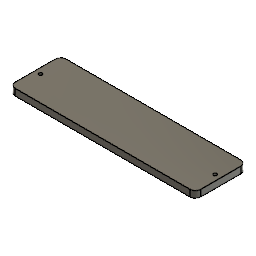
Specimen_Rack_v0 (Autodesk Fusion 360 design; units mm, degrees)
Autodesk Fusion 360 part; units mm, degrees
note: some values were not read from the file. Chosen so that the rebuilt part matches the saved one: which face or edge a step refers to; that a step has no effect; which pieces of a blend or face edit are solid.
sketch "Sketch1" plane through (0, 0, 0) normal (0, 1, 0) x (1, 0, 0) in component "Top_Layer"
  line L0 (0, 0) -> (250, 0)
  line L1 (250, 0) -> (250, 78)
  line L2 (250, 78) -> (0, 78)
  line L3 (0, 78) -> (0, 0)
  line L4 (0, 39) -> (250, 39) construction
  line L5 (0, 78) -> (0, 75) construction
  line L6 (0, 0) -> (0, 3) construction
  line L7 (0, 3) -> (250, 3) construction
  line L8 (0, 75) -> (250, 75) construction
  line L9 (250, 75) -> (247, 75) construction
  line L10 (247, 75) -> (247, 3) construction
  line L11 (0, 3) -> (3, 3) construction
  line L12 (3, 3) -> (3, 75) construction
  circle A0 centre (5.4622, 38.5669) radius 2.5
  circle A1 centre (244.5, 39) radius 2.5
  line L13 (242, 39) -> (237, 39) construction
  line L14 (7.9244, 39) -> (12.9244, 39) construction
  circle A2 centre (211.5, 39) radius 25.5
  circle A3 centre (38.4244, 39) radius 25.5
  line L15 (63.9244, 39) -> (73.9244, 39) construction
  line L16 (186, 39) -> (176, 39) construction
  circle A4 centre (89.4244, 39) radius 15.5
  circle A5 centre (160.5, 39) radius 15.5
  line L17 (104.9244, 39) -> (145, 39) construction
  circle A6 centre (124.9622, 39) radius 15.5
  dimension "d1" = 250
  dimension "d2" = 78
  dimension "d3" = 3
  dimension "d4" = 3
  dimension "d5" = 3
  dimension "d6" = 3
  dimension "d7" = 5
  dimension "d8" = 5
  dimension "d9" = 5
  dimension "d10" = 5
  dimension "d11" = 51
  dimension "d12" = 51
  dimension "d13" = 10
  dimension "d14" = 10
  dimension "d15" = 31
  dimension "d16" = 31
  dimension "d17" = 31
  constraint horizontal L0
  constraint vertical L1
  constraint horizontal L2
  constraint vertical L3
  constraint coincident L0.start L3.end
  constraint midpoint L3 L4.start
  constraint midpoint L1 L4.end
  constraint perpendicular L2 L5
  constraint perpendicular L0 L6
  constraint coincident L1 L7.end
  constraint perpendicular L1 L7
  constraint coincident L1 L8.end
  constraint perpendicular L1 L8
  constraint perpendicular L1 L9
  constraint coincident L7 L10.end
  constraint perpendicular L7 L10
  constraint perpendicular L6 L11
  constraint perpendicular L7 L12
  constraint coincident A1 L13.start
  constraint coincident L4 L13.start
  constraint coincident L4 L13.end
  constraint coincident A0 L14.start
  constraint coincident L4 L14.start
  constraint perpendicular L3 L14
  constraint coincident L13.end A2
  constraint coincident L14.end A3
  constraint coincident A3 L15.start
  constraint coincident L4 L15.start
  constraint parallel L4 L15
  constraint coincident A2 L16.start
  constraint coincident L4 L16.start
  constraint parallel L4 L16
  constraint coincident L15.end A4
  constraint coincident L16.end A5
  constraint coincident A4 L17.start
  constraint coincident L4 L17.start
  constraint coincident A5 L17.end
  constraint coincident L4 L17.end
  constraint midpoint L17 A6.centre
  measures "d1" distance of L0.start L0.end
  measures "d2" distance of L0.start L2.end
  measures "d3" distance of L2.end L5.end
  measures "d4" distance of L0.start L6.end
  measures "d5" distance of L8.end L9.end
  measures "d6" distance of L6.end L11.end
  measures "d7" diameter of A0
  measures "d8" diameter of A1
  measures "d9" distance of L13.start L13.end
  measures "d10" distance of L14.start L14.end
  measures "d11" diameter of A2
  measures "d12" diameter of A3
  measures "d13" distance of L15.start L15.end
  measures "d14" distance of L16.start L16.end
  measures "d15" diameter of A4
  measures "d16" diameter of A5
  measures "d17" diameter of A6
extrude "Extrude1" add sketch "Sketch1" along normal blind 5 contours A0 | A1 makes body 1 at (7.9591, 3.3333, -38.4423) makes body 2 at (245.1771, 3.3333, -41.4066) in component "Top_Layer"
extrude "Extrude2" add sketch "Sketch1" along normal blind 10 bodies 1 2 in component "Top_Layer"
move_face "MoveFace1" to x (1, 0, 0) y (0, 1, 0) z (0, 0, 1) at (50, 0, 0) 2 faces at (250, 3.3333, -26) (245.2962, 6.6667, -41.3698) on bodies 1 in component "Top_Layer"
move_face "MoveFace2" to x (1, 0, 0) y (0, 1, 0) z (0, 0, 1) at (5.462, 0, 0) 2 faces at (175.923, 3.3333, -37.4567) (236.8733, 3.3333, -36.461) on bodies 1 in component "Top_Layer"
move_face "MoveFace3" to x (1, 0, 0) y (0, 1, 0) z (0, 0, 1) at (5.462, 0, 0) 3 faces at (140.4429, 6.6667, -38.2274) (181.385, 3.3333, -37.4567) (242.3353, 3.3333, -36.461) on bodies 1 in component "Top_Layer"
fillet "Fillet1" radius 8 4 edges at (0, 5, -78) (0, 5, 0) (300, 5, 0) (300, 5, -78) on bodies 1 in component "Top_Layer"
sketch "Sketch2" plane through (0, 10, 0) normal (0, 1, 0) x (-1, 0, 0) in component "Top_Layer"
  circle A0 centre (-5.4622, -38.5669) radius 2.5
  circle A1 centre (-38.4244, -39) radius 25.5
  circle A2 centre (-171.424, -39) radius 15.5
  circle A3 centre (-130.4242, -39) radius 15.5
  circle A4 centre (-89.4244, -39) radius 15.5
  circle A5 centre (-294.5, -39) radius 2.5
  circle A6 centre (-222.424, -39) radius 25.5
  arc A7 (-300, -70) -> (-292, -78) centre (-292, -70) ccw
  line L0 (-292, -78) -> (-8, -78)
  arc A8 (-8, -78) -> (0, -70) centre (-8, -70) ccw
  line L1 (0, -70) -> (0, -8)
  arc A9 (0, -8) -> (-8, 0) centre (-8, -8) ccw
  arc A10 (-292, 0) -> (-300, -8) centre (-292, -8) ccw
  line L2 (-300, -8) -> (-300, -70)
  line L3 (-247.9239, -38.9231) -> (-292.0012, -38.9231) construction
  line L4 (-222.424, -39) -> (-171.424, -39) construction
  line L5 (-171.424, -39) -> (-130.4242, -39) construction
  line L6 (-130.4242, -39) -> (-89.4244, -39) construction
  line L7 (-89.4244, -39) -> (-38.4244, -39) construction
  line L8 (-73.9244, -39) -> (-63.9244, -39) construction
  line L9 (-104.9244, -39) -> (-114.9242, -39) construction
  line L10 (-145.9242, -39) -> (-155.924, -39) construction
  line L11 (-186.924, -39) -> (-196.924, -39) construction
  line L12 (-191.924, -39) -> (-191.924, 0) construction
  line L13 (-191.924, 0) -> (-191.924, -6) construction
  line L14 (-68.9244, -39) -> (-68.9244, -78) construction
  line L15 (-68.9244, -78) -> (-68.9244, -72) construction
  line L16 (-191.924, -6) -> (-68.9244, -6) construction
  line L17 (-68.9244, -6) -> (-68.9244, -72) construction
  line L18 (-68.9244, -72) -> (-191.924, -72) construction
  line L19 (-191.924, -72) -> (-191.924, -6) construction
  line L20 (-150.9241, -39) -> (-150.9241, -72) construction
  line L21 (-150.9241, -39) -> (-150.9241, -6) construction
  line L22 (-109.9243, -39) -> (-109.9243, -72) construction
  line L23 (-109.9243, -39) -> (-109.9243, -6) construction
  line L24 (-171.424, -39) -> (-171.424, -23.5) construction
  line L25 (-171.424, -23.5) -> (-171.424, -17.5) construction
  line L26 (-171.424, -17.5) -> (-68.9244, -17.5) construction
  line L27 (-171.424, -39) -> (-171.424, -54.5) construction
  line L28 (-171.424, -54.5) -> (-171.424, -60.5) construction
  line L29 (-171.424, -60.5) -> (-68.9244, -60.4734) construction
  circle A11 centre (-150.9241, -65.5) radius 6.5
  circle A12 centre (-150.9241, -12.5) radius 6.5
  circle A13 centre (-109.9243, -12.5) radius 6.5
  circle A14 centre (-68.9244, -12.5) radius 6.5
  circle A15 centre (-68.9244, -65.5) radius 6.5
  circle A16 centre (-109.926, -65.5) radius 6.5
  circle A17 centre (-191.924, -65.5) radius 6.5
  circle A18 centre (-191.924, -12.5) radius 6.5
  dimension "d32" = 6
  dimension "d33" = 6
  dimension "d34" = 6
  dimension "d35" = 6
  dimension "d36" = 13
  dimension "d37" = 13
  dimension "d38" = 13
  dimension "d39" = 13
  dimension "d40" = 13
  dimension "d41" = 13
  dimension "d42" = 13
  dimension "d43" = 13
  constraint coincident A6 L3.start
  constraint coincident A5 L3.end
  constraint horizontal L3
  constraint coincident A6.centre L4.start
  constraint coincident A2.centre L4.end
  constraint coincident A3.centre L5.end
  constraint coincident A4.centre L6.end
  constraint coincident A1.centre L7.end
  constraint coincident A4 L8.start
  constraint coincident L7 L8.start
  constraint midpoint L7 L8.end
  constraint coincident A4 L9.start
  constraint coincident L6 L9.start
  constraint coincident L6 L9.end
  constraint coincident A3 L9.end
  constraint coincident A3 L10.start
  constraint coincident L5 L10.start
  constraint coincident A2 L10.end
  constraint coincident L5 L10.end
  constraint coincident A2 L11.start
  constraint coincident L4 L11.start
  constraint midpoint L4 L11.end
  constraint midpoint L11 L12.start
  constraint midpoint L8 L14.start
  constraint coincident L0 L14.end
  constraint perpendicular L0 L14
  constraint perpendicular L0 L15
  constraint horizontal L16
  constraint vertical L17
  constraint horizontal L18
  constraint vertical L19
  constraint midpoint L5 L20.start
  constraint coincident L18 L20.end
  constraint perpendicular L18 L20
  constraint coincident L16 L21.end
  constraint perpendicular L16 L21
  constraint midpoint L6 L22.start
  constraint coincident L18 L22.end
  constraint perpendicular L18 L22
  constraint coincident L16 L23.end
  constraint perpendicular L16 L23
  constraint coincident A2 L24.end
  constraint perpendicular L4 L24
  constraint parallel L24 L25
  constraint coincident L17 L26.end
  constraint perpendicular L17 L26
  constraint coincident A2 L27.end
  constraint perpendicular L4 L27
  constraint parallel L27 L28
  constraint coincident L17 L29.end
  constraint coincident L20.end A11
  constraint coincident L21.end A12
  constraint coincident L23.end A13
  constraint coincident L16.end A14
  constraint coincident L15.end A15
  constraint coincident L22.end A16
  constraint coincident L18.end A17
  constraint coincident L13.end A18
  measures "d32" distance of L12.end L13.end
  measures "d33" distance of L14.end L15.end
  measures "d34" distance of L24.end L25.end
  measures "d35" distance of L27.end L28.end
  measures "d36" diameter of A11
  measures "d37" diameter of A12
  measures "d38" diameter of A13
  measures "d39" diameter of A14
  measures "d40" diameter of A15
  measures "d41" diameter of A16
  measures "d42" diameter of A17
  measures "d43" diameter of A18
extrude "Extrude3" cut sketch "Sketch2" against normal blind 10 contours A11 | A12 | A13 | A14 | A15 | A16 | A17 | A18 bodies 1 in component "Top_Layer"
sketch "Sketch3" plane through (0, 10, 0) normal (0, 1, 0) x (-1, 0, 0) in component "Top_Layer"
move_face "MoveFace4" to x (1, 0, 0) y (0, 1, 0) z (0, 0, 1) at (-34.07, 0, 0) 7 faces at (282.6413, 0, -39) (297.7899, 6.6667, -75.5206) (276.6758, 10, -56.2406) (300, 3.3333, -28.6667) (297.7899, 3.3333, -2.4794) (294.9341, 6.6667, -41.462) (295.1109, 5, -38.1848) on bodies 1 in component "Top_Layer"
move_face "MoveFace5" to x (1, 0, 0) y (0, 1, 0) z (0, 0, 1) at (-0.006, 0, 0) 2 faces at (265.93, 3.3333, -28.6667) (260.7409, 8.3333, -41.4806) on bodies 1 in component "Top_Layer"
move_face "MoveFace6" by (3, 0, 0) 1 faces at (265.93, 3.3333, -28.6667) on bodies 1 in component "Top_Layer"
move_face "MoveFace7" to x (1, 0, 0) y (0, 1, 0) z (0, 0, 1) at (-5.025, 0, 0) 5 faces at (0.0091, 3.3333, -70.3807) (7.6193, 3.3333, -0.0091) (0, 3.3333, -49.3333) (7.9591, 6.6667, -38.6915) (4.6036, 5, -39.1523) on bodies 1 in component "Top_Layer"
move_face "MoveFace8" to x (1, 0, 0) y (0, 1, 0) z (0, 0, 1) at (-0.005, 0, 0) 2 faces at (2.9341, 6.6667, -38.6915) (-5.025, 5, -64.039) on bodies 1 in component "Top_Layer"
move_face "MoveFace9" by (-3.038, 0, 0) 1 faces at (-5.025, 5, -64.039) on bodies 1 in component "Top_Layer"
sketch "Sketch4" plane through (0, 10, 0) normal (0, 1, 0) x (-1, 0, 0) in component "Top_Layer"
  arc A0 (8.068, -8) -> (0.068, 0) centre (0.068, -8) ccw
  line L0 (0.068, 0) -> (-260.924, 0)
  arc A1 (-260.924, 0) -> (-268.924, -8) centre (-260.924, -8) ccw
  line L1 (-268.924, -8) -> (-268.924, -70)
  arc A2 (-268.924, -70) -> (-260.924, -78) centre (-260.924, -70) ccw
  line L2 (-260.924, -78) -> (0.068, -78)
  arc A3 (0.068, -78) -> (8.068, -70) centre (0.068, -70) ccw
  line L3 (8.068, -70) -> (8.068, -8)
  circle A4 centre (-109.9243, -12.5) radius 6.5
  circle A5 centre (-191.924, -12.5) radius 6.5
  circle A6 centre (-150.9241, -12.5) radius 6.5
  circle A7 centre (-68.9244, -12.5) radius 6.5
  circle A8 centre (-150.9241, -65.5) radius 6.5
  circle A9 centre (-191.924, -65.5) radius 6.5
  circle A10 centre (-109.926, -65.5) radius 6.5
  circle A11 centre (-68.9244, -65.5) radius 6.5
  circle A12 centre (-0.4322, -38.5669) radius 2.5
  circle A13 centre (-38.4244, -39) radius 25.5
  circle A14 centre (-171.424, -39) radius 15.5
  circle A15 centre (-130.4242, -39) radius 15.5
  circle A16 centre (-89.4244, -39) radius 15.5
  circle A17 centre (-260.424, -39) radius 2.5
  circle A18 centre (-222.424, -39) radius 25.5
  line L4 (-260.424, -39) -> (-247.924, -39) construction
  line L5 (-191.924, -65.5) -> (-191.924, -72) construction
  line L6 (-191.924, -72) -> (-268.67, -72) construction
  line L7 (-254.174, -39) -> (-254.174, -72) construction
  line L8 (-254.174, -39) -> (-191.9575, -39) construction
  line L9 (-191.9575, -39) -> (-191.9575, -6.0001) construction
  line L10 (-191.9575, -6.0001) -> (-254.174, -6.0001) construction
  line L11 (-254.174, -6.0001) -> (-254.174, -39) construction
  circle A19 centre (-254.174, -12.5001) radius 6.5
  circle A20 centre (-254.174, -65.5) radius 6.5
  dimension "d64" = 13
  dimension "d65" = 13
  constraint coincident A17.centre L4.start
  constraint coincident A18 L4.end
  constraint perpendicular L1 L4
  constraint coincident A9.centre L5.start
  constraint coincident A9 L5.end
  constraint vertical L5
  constraint coincident A2 L6.end
  constraint tangent A9 L6
  constraint midpoint L4 L7.start
  constraint coincident L6 L7.end
  constraint perpendicular L6 L7
  constraint horizontal L8
  constraint vertical L9
  constraint horizontal L10
  constraint vertical L11
  constraint coincident A5 L9.end
  constraint coincident L10.end A19
  constraint coincident L7.end A20
  measures "d64" diameter of A19
  measures "d65" diameter of A20
extrude "Extrude4" cut sketch "Sketch4" against normal blind 13 contours A19 | A20 bodies 1 in component "Top_Layer"
sketch "Sketch5" plane through (0, 10, 0) normal (0, 1, 0) x (-1, 0, 0) in component "Top_Layer"
  circle A0 centre (-254.174, -65.5) radius 6.5
  circle A1 centre (-254.174, -12.5001) radius 6.5
  arc A2 (8.068, -8) -> (0.068, 0) centre (0.068, -8) ccw
  line L0 (0.068, 0) -> (-260.924, 0)
  arc A3 (-260.924, 0) -> (-268.924, -8) centre (-260.924, -8) ccw
  line L1 (-268.924, -8) -> (-268.924, -70)
  arc A4 (-268.924, -70) -> (-260.924, -78) centre (-260.924, -70) ccw
  line L2 (-260.924, -78) -> (0.068, -78)
  arc A5 (0.068, -78) -> (8.068, -70) centre (0.068, -70) ccw
  line L3 (8.068, -70) -> (8.068, -8)
  circle A6 centre (-109.9243, -12.5) radius 6.5
  circle A7 centre (-191.924, -12.5) radius 6.5
  circle A8 centre (-150.9241, -12.5) radius 6.5
  circle A9 centre (-68.9244, -12.5) radius 6.5
  circle A10 centre (-150.9241, -65.5) radius 6.5
  circle A11 centre (-191.924, -65.5) radius 6.5
  circle A12 centre (-109.926, -65.5) radius 6.5
  circle A13 centre (-68.9244, -65.5) radius 6.5
  circle A14 centre (-0.4322, -38.5669) radius 2.5
  circle A15 centre (-38.4244, -39) radius 25.5
  circle A16 centre (-171.424, -39) radius 15.5
  circle A17 centre (-130.4242, -39) radius 15.5
  circle A18 centre (-89.4244, -39) radius 15.5
  circle A19 centre (-260.424, -39) radius 2.5
  circle A20 centre (-222.424, -39) radius 25.5
  line L4 (-0.4322, -38.5669) -> (-2.9322, -38.5669) construction
  line L5 (-2.9322, -38.5669) -> (-12.9281, -38.5669) construction
  line L6 (-69.0119, -6.0006) -> (-66.2573, -5.9635) construction
  line L7 (-66.2573, -5.9635) -> (7.8045, -5.9635) construction
  line L8 (-7.9301, -38.5669) -> (-7.9301, -5.9635) construction
  line L9 (-7.9301, -5.9635) -> (-68.6986, -5.9635) construction
  line L10 (-68.6986, -5.9635) -> (-68.6986, -71.9961) construction
  line L11 (-68.6986, -71.9961) -> (-7.9301, -71.9961) construction
  line L12 (-7.9301, -71.9961) -> (-7.9301, -5.9635) construction
  circle A21 centre (-7.9301, -12.4635) radius 6.5
  circle A22 centre (-7.9301, -65.4961) radius 6.5
  dimension "d68" = 13
  dimension "d69" = 13
  constraint coincident A14.centre L4.start
  constraint coincident A14 L4.end
  constraint horizontal L4
  constraint coincident A15 L5.end
  constraint parallel L4 L5
  constraint coincident A9 L6.start
  constraint tangent A9 L6
  constraint coincident A2 L7.end
  constraint parallel L0 L7
  constraint midpoint L5 L8.start
  constraint coincident L7 L8.end
  constraint perpendicular L7 L8
  constraint horizontal L9
  constraint vertical L10
  constraint horizontal L11
  constraint vertical L12
  constraint coincident A13 L10.end
  constraint coincident L8.end A21
  constraint coincident L11.end A22
  measures "d68" diameter of A21
  measures "d69" diameter of A22
extrude "Extrude5" cut sketch "Sketch5" against normal blind 10 contours A21 | A22 bodies 1 in component "Top_Layer"
move_face "MoveFace10" to x (1, 0, 0) y (0, 1, 0) z (0, 0, 1) at (0, 0, 2) 6 faces at (1.4382, 3.3333, -65.8201) (62.4325, 3.3333, -65.824) (103.4341, 3.3333, -65.824) (144.4322, 3.3333, -65.824) (185.4563, 6.6667, -66.1472) (258.475, 6.6667, -60.6264) on bodies 1 in component "Top_Layer"
move_face "MoveFace11" to x (1, 0, 0) y (0, 1, 0) z (0, 0, 1) at (0, 0, -2) 6 faces at (1.4382, 3.3333, -12.7875) (62.4325, 3.3333, -12.824) (103.4324, 3.3333, -12.824) (144.4322, 3.3333, -12.824) (185.4563, 6.6667, -13.1472) (258.475, 6.6667, -7.6265) on bodies 1 in component "Top_Layer"
sketch "Sketch1 (2)" plane through (0, 0, 0) normal (0, 1, 0) x (1, 0, 0) in component "Bottom_Layer"
  line L0 (0, 0) -> (250, 0)
  line L1 (250, 0) -> (250, 78)
  line L2 (250, 78) -> (0, 78)
  line L3 (0, 78) -> (0, 0)
  line L4 (0, 39) -> (250, 39) construction
  line L5 (0, 78) -> (0, 75) construction
  line L6 (0, 0) -> (0, 3) construction
  line L7 (0, 3) -> (250, 3) construction
  line L8 (0, 75) -> (250, 75) construction
  line L9 (250, 75) -> (247, 75) construction
  line L10 (247, 75) -> (247, 3) construction
  line L11 (0, 3) -> (3, 3) construction
  line L12 (3, 3) -> (3, 75) construction
  circle A0 centre (5.4622, 38.5669) radius 2.5
  circle A1 centre (244.5, 39) radius 2.5
  line L13 (242, 39) -> (237, 39) construction
  line L14 (7.9244, 39) -> (12.9244, 39) construction
  circle A2 centre (211.5, 39) radius 25.5
  circle A3 centre (38.4244, 39) radius 25.5
  line L15 (63.9244, 39) -> (73.9244, 39) construction
  line L16 (186, 39) -> (176, 39) construction
  circle A4 centre (89.4244, 39) radius 15.5
  circle A5 centre (160.5, 39) radius 15.5
  line L17 (104.9244, 39) -> (145, 39) construction
  circle A6 centre (124.9622, 39) radius 15.5
  dimension "d1_1" = 250
  dimension "d2_1" = 78
  dimension "d3_1" = 3
  dimension "d4_1" = 3
  dimension "d5_1" = 3
  dimension "d6_1" = 3
  dimension "d7_1" = 5
  dimension "d8_1" = 5
  dimension "d9_1" = 5
  dimension "d10_1" = 5
  dimension "d11_1" = 51
  dimension "d12_1" = 51
  dimension "d13_1" = 10
  dimension "d14_1" = 10
  dimension "d15_1" = 31
  dimension "d16_1" = 31
  dimension "d17_1" = 31
  constraint horizontal L0
  constraint vertical L1
  constraint horizontal L2
  constraint vertical L3
  constraint coincident L0.start L3.end
  constraint midpoint L3 L4.start
  constraint midpoint L1 L4.end
  constraint perpendicular L2 L5
  constraint perpendicular L0 L6
  constraint coincident L1 L7.end
  constraint perpendicular L1 L7
  constraint coincident L1 L8.end
  constraint perpendicular L1 L8
  constraint perpendicular L1 L9
  constraint coincident L7 L10.end
  constraint perpendicular L7 L10
  constraint perpendicular L6 L11
  constraint perpendicular L7 L12
  constraint coincident A1 L13.start
  constraint coincident L4 L13.start
  constraint coincident L4 L13.end
  constraint coincident A0 L14.start
  constraint coincident L4 L14.start
  constraint perpendicular L3 L14
  constraint coincident L13.end A2
  constraint coincident L14.end A3
  constraint coincident A3 L15.start
  constraint coincident L4 L15.start
  constraint parallel L4 L15
  constraint coincident A2 L16.start
  constraint coincident L4 L16.start
  constraint parallel L4 L16
  constraint coincident L15.end A4
  constraint coincident L16.end A5
  constraint coincident A4 L17.start
  constraint coincident L4 L17.start
  constraint coincident A5 L17.end
  constraint coincident L4 L17.end
  constraint midpoint L17 A6.centre
  measures "d1_1" distance of L0.start L0.end
  measures "d2_1" distance of L0.start L2.end
  measures "d3_1" distance of L2.end L5.end
  measures "d4_1" distance of L0.start L6.end
  measures "d5_1" distance of L8.end L9.end
  measures "d6_1" distance of L6.end L11.end
  measures "d7_1" diameter of A0
  measures "d8_1" diameter of A1
  measures "d9_1" distance of L13.start L13.end
  measures "d10_1" distance of L14.start L14.end
  measures "d11_1" diameter of A2
  measures "d12_1" diameter of A3
  measures "d13_1" distance of L15.start L15.end
  measures "d14_1" distance of L16.start L16.end
  measures "d15_1" diameter of A4
  measures "d16_1" diameter of A5
  measures "d17_1" diameter of A6
extrude "Extrude1'" add sketch "Sketch1 (2)" along normal blind 5 separate body contours A0 | A1 makes body 3 at (7.9591, 3.3333, -38.4423) makes body 4 at (245.1771, 3.3333, -41.4066) in component "Bottom_Layer"
extrude "Extrude2'" add sketch "Sketch1 (2)" along normal blind 10 bodies 3 4 in component "Bottom_Layer"
move_face "MoveFace1'" to x (1, 0, 0) y (0, 1, 0) z (0, 0, 1) at (50, 0, 0) 2 faces at (250, 3.3333, -26) (245.2962, 6.6667, -41.3698) on bodies 3 in component "Bottom_Layer"
move_face "MoveFace2'" to x (1, 0, 0) y (0, 1, 0) z (0, 0, 1) at (5.462, 0, 0) 2 faces at (175.923, 3.3333, -37.4567) (236.8733, 3.3333, -36.461) on bodies 3 in component "Bottom_Layer"
move_face "MoveFace3'" to x (1, 0, 0) y (0, 1, 0) z (0, 0, 1) at (5.462, 0, 0) 3 faces at (140.4429, 6.6667, -38.2274) (181.385, 3.3333, -37.4567) (242.3353, 3.3333, -36.461) on bodies 3 in component "Bottom_Layer"
fillet "Fillet1'" radius 8 4 edges at (0, 5, -78) (0, 5, 0) (300, 5, 0) (300, 5, -78) on bodies 3 in component "Bottom_Layer"
sketch "Sketch2 (2)" plane through (0, 10, 0) normal (0, 1, 0) x (-1, 0, 0) in component "Bottom_Layer"
  circle A0 centre (-5.4622, -38.5669) radius 2.5
  circle A1 centre (-38.4244, -39) radius 25.5
  circle A2 centre (-171.424, -39) radius 15.5
  circle A3 centre (-130.4242, -39) radius 15.5
  circle A4 centre (-89.4244, -39) radius 15.5
  circle A5 centre (-294.5, -39) radius 2.5
  circle A6 centre (-222.424, -39) radius 25.5
  arc A7 (-300, -70) -> (-292, -78) centre (-292, -70) ccw
  line L0 (-292, -78) -> (-8, -78)
  arc A8 (-8, -78) -> (0, -70) centre (-8, -70) ccw
  line L1 (0, -70) -> (0, -8)
  arc A9 (0, -8) -> (-8, 0) centre (-8, -8) ccw
  arc A10 (-292, 0) -> (-300, -8) centre (-292, -8) ccw
  line L2 (-300, -8) -> (-300, -70)
  line L3 (-247.9239, -38.9231) -> (-292.0012, -38.9231) construction
  line L4 (-222.424, -39) -> (-171.424, -39) construction
  line L5 (-171.424, -39) -> (-130.4242, -39) construction
  line L6 (-130.4242, -39) -> (-89.4244, -39) construction
  line L7 (-89.4244, -39) -> (-38.4244, -39) construction
  line L8 (-73.9244, -39) -> (-63.9244, -39) construction
  line L9 (-104.9244, -39) -> (-114.9242, -39) construction
  line L10 (-145.9242, -39) -> (-155.924, -39) construction
  line L11 (-186.924, -39) -> (-196.924, -39) construction
  line L12 (-191.924, -39) -> (-191.924, 0) construction
  line L13 (-191.924, 0) -> (-191.924, -6) construction
  line L14 (-68.9244, -39) -> (-68.9244, -78) construction
  line L15 (-68.9244, -78) -> (-68.9244, -72) construction
  line L16 (-191.924, -6) -> (-68.9244, -6) construction
  line L17 (-68.9244, -6) -> (-68.9244, -72) construction
  line L18 (-68.9244, -72) -> (-191.924, -72) construction
  line L19 (-191.924, -72) -> (-191.924, -6) construction
  line L20 (-150.9241, -39) -> (-150.9241, -72) construction
  line L21 (-150.9241, -39) -> (-150.9241, -6) construction
  line L22 (-109.9243, -39) -> (-109.9243, -72) construction
  line L23 (-109.9243, -39) -> (-109.9243, -6) construction
  line L24 (-171.424, -39) -> (-171.424, -23.5) construction
  line L25 (-171.424, -23.5) -> (-171.424, -17.5) construction
  line L26 (-171.424, -17.5) -> (-68.9244, -17.5) construction
  line L27 (-171.424, -39) -> (-171.424, -54.5) construction
  line L28 (-171.424, -54.5) -> (-171.424, -60.5) construction
  line L29 (-171.424, -60.5) -> (-68.9244, -60.4734) construction
  circle A11 centre (-150.9241, -65.5) radius 6.5
  circle A12 centre (-150.9241, -12.5) radius 6.5
  circle A13 centre (-109.9243, -12.5) radius 6.5
  circle A14 centre (-68.9244, -12.5) radius 6.5
  circle A15 centre (-68.9244, -65.5) radius 6.5
  circle A16 centre (-109.926, -65.5) radius 6.5
  circle A17 centre (-191.924, -65.5) radius 6.5
  circle A18 centre (-191.924, -12.5) radius 6.5
  dimension "d32_1" = 6
  dimension "d33_1" = 6
  dimension "d34_1" = 6
  dimension "d35_1" = 6
  dimension "d36_1" = 13
  dimension "d37_1" = 13
  dimension "d38_1" = 13
  dimension "d39_1" = 13
  dimension "d40_1" = 13
  dimension "d41_1" = 13
  dimension "d42_1" = 13
  dimension "d43_1" = 13
  constraint coincident A6 L3.start
  constraint coincident A5 L3.end
  constraint horizontal L3
  constraint coincident A6.centre L4.start
  constraint coincident A2.centre L4.end
  constraint coincident A3.centre L5.end
  constraint coincident A4.centre L6.end
  constraint coincident A1.centre L7.end
  constraint coincident A4 L8.start
  constraint coincident L7 L8.start
  constraint midpoint L7 L8.end
  constraint coincident A4 L9.start
  constraint coincident L6 L9.start
  constraint coincident L6 L9.end
  constraint coincident A3 L9.end
  constraint coincident A3 L10.start
  constraint coincident L5 L10.start
  constraint coincident A2 L10.end
  constraint coincident L5 L10.end
  constraint coincident A2 L11.start
  constraint coincident L4 L11.start
  constraint midpoint L4 L11.end
  constraint midpoint L11 L12.start
  constraint midpoint L8 L14.start
  constraint coincident L0 L14.end
  constraint perpendicular L0 L14
  constraint perpendicular L0 L15
  constraint horizontal L16
  constraint vertical L17
  constraint horizontal L18
  constraint vertical L19
  constraint midpoint L5 L20.start
  constraint coincident L18 L20.end
  constraint perpendicular L18 L20
  constraint coincident L16 L21.end
  constraint perpendicular L16 L21
  constraint midpoint L6 L22.start
  constraint coincident L18 L22.end
  constraint perpendicular L18 L22
  constraint coincident L16 L23.end
  constraint perpendicular L16 L23
  constraint coincident A2 L24.end
  constraint perpendicular L4 L24
  constraint parallel L24 L25
  constraint coincident L17 L26.end
  constraint perpendicular L17 L26
  constraint coincident A2 L27.end
  constraint perpendicular L4 L27
  constraint parallel L27 L28
  constraint coincident L17 L29.end
  constraint coincident L20.end A11
  constraint coincident L21.end A12
  constraint coincident L23.end A13
  constraint coincident L16.end A14
  constraint coincident L15.end A15
  constraint coincident L22.end A16
  constraint coincident L18.end A17
  constraint coincident L13.end A18
  measures "d32_1" distance of L12.end L13.end
  measures "d33_1" distance of L14.end L15.end
  measures "d34_1" distance of L24.end L25.end
  measures "d35_1" distance of L27.end L28.end
  measures "d36_1" diameter of A11
  measures "d37_1" diameter of A12
  measures "d38_1" diameter of A13
  measures "d39_1" diameter of A14
  measures "d40_1" diameter of A15
  measures "d41_1" diameter of A16
  measures "d42_1" diameter of A17
  measures "d43_1" diameter of A18
extrude "Extrude3'" cut sketch "Sketch2 (2)" against normal blind 10 contours A11 | A12 | A13 | A14 | A15 | A16 | A17 | A18 bodies 3 in component "Bottom_Layer"
sketch "Sketch3 (2)" plane through (0, 10, 0) normal (0, 1, 0) x (-1, 0, 0) in component "Bottom_Layer"
move_face "MoveFace4'" to x (1, 0, 0) y (0, 1, 0) z (0, 0, 1) at (-34.07, 0, 0) 7 faces at (282.6413, 0, -39) (297.7899, 6.6667, -75.5206) (276.6758, 10, -56.2406) (300, 3.3333, -28.6667) (297.7899, 3.3333, -2.4794) (294.9341, 6.6667, -41.462) (295.1109, 5, -38.1848) on bodies 3 in component "Bottom_Layer"
move_face "MoveFace5'" to x (1, 0, 0) y (0, 1, 0) z (0, 0, 1) at (-0.006, 0, 0) 2 faces at (265.93, 3.3333, -28.6667) (260.7409, 8.3333, -41.4806) on bodies 3 in component "Bottom_Layer"
move_face "MoveFace6'" by (3, 0, 0) 1 faces at (265.93, 3.3333, -28.6667) on bodies 3 in component "Bottom_Layer"
move_face "MoveFace7'" to x (1, 0, 0) y (0, 1, 0) z (0, 0, 1) at (-5.025, 0, 0) 5 faces at (0.0091, 3.3333, -70.3807) (7.6193, 3.3333, -0.0091) (0, 3.3333, -49.3333) (7.9591, 6.6667, -38.6915) (4.6036, 5, -39.1523) on bodies 3 in component "Bottom_Layer"
move_face "MoveFace8'" to x (1, 0, 0) y (0, 1, 0) z (0, 0, 1) at (-0.005, 0, 0) 2 faces at (2.9341, 6.6667, -38.6915) (-5.025, 5, -64.039) on bodies 3 in component "Bottom_Layer"
move_face "MoveFace9'" by (-3.038, 0, 0) 1 faces at (-5.025, 5, -64.039) on bodies 3 in component "Bottom_Layer"
sketch "Sketch4 (2)" plane through (0, 10, 0) normal (0, 1, 0) x (-1, 0, 0) in component "Bottom_Layer"
  arc A0 (8.068, -8) -> (0.068, 0) centre (0.068, -8) ccw
  line L0 (0.068, 0) -> (-260.924, 0)
  arc A1 (-260.924, 0) -> (-268.924, -8) centre (-260.924, -8) ccw
  line L1 (-268.924, -8) -> (-268.924, -70)
  arc A2 (-268.924, -70) -> (-260.924, -78) centre (-260.924, -70) ccw
  line L2 (-260.924, -78) -> (0.068, -78)
  arc A3 (0.068, -78) -> (8.068, -70) centre (0.068, -70) ccw
  line L3 (8.068, -70) -> (8.068, -8)
  circle A4 centre (-109.9243, -12.5) radius 6.5
  circle A5 centre (-191.924, -12.5) radius 6.5
  circle A6 centre (-150.9241, -12.5) radius 6.5
  circle A7 centre (-68.9244, -12.5) radius 6.5
  circle A8 centre (-150.9241, -65.5) radius 6.5
  circle A9 centre (-191.924, -65.5) radius 6.5
  circle A10 centre (-109.926, -65.5) radius 6.5
  circle A11 centre (-68.9244, -65.5) radius 6.5
  circle A12 centre (-0.4322, -38.5669) radius 2.5
  circle A13 centre (-38.4244, -39) radius 25.5
  circle A14 centre (-171.424, -39) radius 15.5
  circle A15 centre (-130.4242, -39) radius 15.5
  circle A16 centre (-89.4244, -39) radius 15.5
  circle A17 centre (-260.424, -39) radius 2.5
  circle A18 centre (-222.424, -39) radius 25.5
  line L4 (-260.424, -39) -> (-247.924, -39) construction
  line L5 (-191.924, -65.5) -> (-191.924, -72) construction
  line L6 (-191.924, -72) -> (-268.67, -72) construction
  line L7 (-254.174, -39) -> (-254.174, -72) construction
  line L8 (-254.174, -39) -> (-191.9575, -39) construction
  line L9 (-191.9575, -39) -> (-191.9575, -6.0001) construction
  line L10 (-191.9575, -6.0001) -> (-254.174, -6.0001) construction
  line L11 (-254.174, -6.0001) -> (-254.174, -39) construction
  circle A19 centre (-254.174, -12.5001) radius 6.5
  circle A20 centre (-254.174, -65.5) radius 6.5
  dimension "d64_1" = 13
  dimension "d65_1" = 13
  constraint coincident A17.centre L4.start
  constraint coincident A18 L4.end
  constraint perpendicular L1 L4
  constraint coincident A9.centre L5.start
  constraint coincident A9 L5.end
  constraint vertical L5
  constraint coincident A2 L6.end
  constraint tangent A9 L6
  constraint midpoint L4 L7.start
  constraint coincident L6 L7.end
  constraint perpendicular L6 L7
  constraint horizontal L8
  constraint vertical L9
  constraint horizontal L10
  constraint vertical L11
  constraint coincident A5 L9.end
  constraint coincident L10.end A19
  constraint coincident L7.end A20
  measures "d64_1" diameter of A19
  measures "d65_1" diameter of A20
extrude "Extrude4'" cut sketch "Sketch4 (2)" against normal blind 13 contours A19 | A20 bodies 3 in component "Bottom_Layer"
sketch "Sketch5 (2)" plane through (0, 10, 0) normal (0, 1, 0) x (-1, 0, 0) in component "Bottom_Layer"
  circle A0 centre (-254.174, -65.5) radius 6.5
  circle A1 centre (-254.174, -12.5001) radius 6.5
  arc A2 (8.068, -8) -> (0.068, 0) centre (0.068, -8) ccw
  line L0 (0.068, 0) -> (-260.924, 0)
  arc A3 (-260.924, 0) -> (-268.924, -8) centre (-260.924, -8) ccw
  line L1 (-268.924, -8) -> (-268.924, -70)
  arc A4 (-268.924, -70) -> (-260.924, -78) centre (-260.924, -70) ccw
  line L2 (-260.924, -78) -> (0.068, -78)
  arc A5 (0.068, -78) -> (8.068, -70) centre (0.068, -70) ccw
  line L3 (8.068, -70) -> (8.068, -8)
  circle A6 centre (-109.9243, -12.5) radius 6.5
  circle A7 centre (-191.924, -12.5) radius 6.5
  circle A8 centre (-150.9241, -12.5) radius 6.5
  circle A9 centre (-68.9244, -12.5) radius 6.5
  circle A10 centre (-150.9241, -65.5) radius 6.5
  circle A11 centre (-191.924, -65.5) radius 6.5
  circle A12 centre (-109.926, -65.5) radius 6.5
  circle A13 centre (-68.9244, -65.5) radius 6.5
  circle A14 centre (-0.4322, -38.5669) radius 2.5
  circle A15 centre (-38.4244, -39) radius 25.5
  circle A16 centre (-171.424, -39) radius 15.5
  circle A17 centre (-130.4242, -39) radius 15.5
  circle A18 centre (-89.4244, -39) radius 15.5
  circle A19 centre (-260.424, -39) radius 2.5
  circle A20 centre (-222.424, -39) radius 25.5
  line L4 (-0.4322, -38.5669) -> (-2.9322, -38.5669) construction
  line L5 (-2.9322, -38.5669) -> (-12.9281, -38.5669) construction
  line L6 (-69.0119, -6.0006) -> (-66.2573, -5.9635) construction
  line L7 (-66.2573, -5.9635) -> (7.8045, -5.9635) construction
  line L8 (-7.9301, -38.5669) -> (-7.9301, -5.9635) construction
  line L9 (-7.9301, -5.9635) -> (-68.6986, -5.9635) construction
  line L10 (-68.6986, -5.9635) -> (-68.6986, -71.9961) construction
  line L11 (-68.6986, -71.9961) -> (-7.9301, -71.9961) construction
  line L12 (-7.9301, -71.9961) -> (-7.9301, -5.9635) construction
  circle A21 centre (-7.9301, -12.4635) radius 6.5
  circle A22 centre (-7.9301, -65.4961) radius 6.5
  dimension "d68_1" = 13
  dimension "d69_1" = 13
  constraint coincident A14.centre L4.start
  constraint coincident A14 L4.end
  constraint horizontal L4
  constraint coincident A15 L5.end
  constraint parallel L4 L5
  constraint coincident A9 L6.start
  constraint tangent A9 L6
  constraint coincident A2 L7.end
  constraint parallel L0 L7
  constraint midpoint L5 L8.start
  constraint coincident L7 L8.end
  constraint perpendicular L7 L8
  constraint horizontal L9
  constraint vertical L10
  constraint horizontal L11
  constraint vertical L12
  constraint coincident A13 L10.end
  constraint coincident L8.end A21
  constraint coincident L11.end A22
  measures "d68_1" diameter of A21
  measures "d69_1" diameter of A22
extrude "Extrude5'" cut sketch "Sketch5 (2)" against normal blind 10 contours A21 | A22 bodies 3 in component "Bottom_Layer"
move_face "MoveFace10'" to x (1, 0, 0) y (0, 1, 0) z (0, 0, 1) at (0, 0, 2) 6 faces at (1.4382, 3.3333, -65.8201) (62.4325, 3.3333, -65.824) (103.4341, 3.3333, -65.824) (144.4322, 3.3333, -65.824) (185.4563, 6.6667, -66.1472) (258.475, 6.6667, -60.6264) on bodies 3 in component "Bottom_Layer"
move_face "MoveFace11'" to x (1, 0, 0) y (0, 1, 0) z (0, 0, 1) at (0, 0, -2) 6 faces at (1.4382, 3.3333, -12.7875) (62.4325, 3.3333, -12.824) (103.4324, 3.3333, -12.824) (144.4322, 3.3333, -12.824) (185.4563, 6.6667, -13.1472) (258.475, 6.6667, -7.6265) on bodies 3 in component "Bottom_Layer"
delete_face "DeleteFace1" 17 faces at (247.8923, 3.3333, -40.2711) (185.4563, 6.6667, -64.1472) (258.475, 6.6667, -58.6264) (258.475, 6.6667, -9.6265) (185.4563, 6.6667, -15.1472) (144.4322, 3.3333, -14.824) (186.9047, 3.3333, -39.7726) (145.9049, 3.3333, -39.7726) (144.4322, 3.3333, -63.824) (103.4341, 3.3333, -63.824) (103.4324, 3.3333, -14.824) (104.9051, 3.3333, -39.7726) (62.4325, 3.3333, -14.824) (62.4325, 3.3333, -63.824) (63.8927, 3.3333, -40.2711) (1.4382, 3.3333, -14.7875) (1.4382, 3.3333, -63.8201) on bodies 3 in component "Bottom_Layer"
move_face "MoveFace12" by (0, 0, -1) 1 faces at (173.9323, 6.6667, 0) on bodies 1 in component "Top_Layer"
move_face "MoveFace13" by (0, 0, 1) 1 faces at (173.9323, 3.3333, -78) on bodies 1 in component "Top_Layer"
move_face "OffsetFaces1" offset -0.75 1 faces at (1.4382, 3.3333, -14.7875) on bodies 1 in component "Top_Layer"
move_face "OffsetFaces2" offset -0.75 1 faces at (1.4382, 3.3333, -63.8201) on bodies 1 in component "Top_Layer"
move_face "OffsetFaces3" offset -0.75 1 faces at (62.4325, 3.3333, -63.824) on bodies 1 in component "Top_Layer"
move_face "OffsetFaces4" offset -0.75 1 faces at (62.4325, 3.3333, -14.824) on bodies 1 in component "Top_Layer"
move_face "OffsetFaces5" offset -0.75 1 faces at (103.4324, 3.3333, -14.824) on bodies 1 in component "Top_Layer"
move_face "OffsetFaces6" offset -0.75 1 faces at (103.4341, 3.3333, -63.824) on bodies 1 in component "Top_Layer"
move_face "OffsetFaces7" offset -0.75 1 faces at (144.4322, 3.3333, -63.824) on bodies 1 in component "Top_Layer"
move_face "OffsetFaces8" offset -0.75 1 faces at (144.4322, 3.3333, -14.824) on bodies 1 in component "Top_Layer"
move_face "OffsetFaces9" offset -0.75 1 faces at (185.4321, 3.3333, -14.824) on bodies 1 in component "Top_Layer"
move_face "OffsetFaces10" offset -0.75 1 faces at (185.4321, 3.3333, -63.824) on bodies 1 in component "Top_Layer"
move_face "OffsetFaces11" offset -0.75 1 faces at (258.7125, 3.3333, -58.8469) on bodies 1 in component "Top_Layer"
move_face "OffsetFaces12" offset -0.75 1 faces at (258.7125, 3.3333, -9.847) on bodies 1 in component "Top_Layer"
move_face "MoveFace12'" by (0, 0, -1) 1 faces at (173.9323, 6.6667, 0) on bodies 3 in component "Bottom_Layer"
move_face "MoveFace13'" by (0, 0, 1) 1 faces at (173.9323, 3.3333, -78) on bodies 3 in component "Bottom_Layer"
sketch "Sketch6" plane through (0, 10, 0) normal (0, 1, 0) x (-1, 0, 0) in component "Top_Layer"
  arc A0 (-268.924, -69) -> (-260.924, -77) centre (-260.924, -69) ccw
  line L0 (-260.924, -77) -> (0.068, -77)
  arc A1 (0.068, -77) -> (8.068, -69) centre (0.068, -69) ccw
  line L1 (8.068, -69) -> (8.068, -9)
  arc A2 (8.068, -9) -> (0.068, -1) centre (0.068, -9) ccw
  line L2 (0.068, -1) -> (-260.924, -1)
  arc A3 (-260.924, -1) -> (-268.924, -9) centre (-260.924, -9) ccw
  line L3 (-268.924, -9) -> (-268.924, -69)
  circle A4 centre (-7.9301, -63.4961) radius 7.25
  circle A5 centre (-7.9301, -14.4635) radius 7.25
  circle A6 centre (-254.174, -63.5) radius 7.25
  circle A7 centre (-254.174, -14.5001) radius 7.25
  circle A8 centre (-109.9243, -14.5) radius 7.25
  circle A9 centre (-191.924, -14.5) radius 7.25
  circle A10 centre (-150.9241, -14.5) radius 7.25
  circle A11 centre (-68.9244, -14.5) radius 7.25
  circle A12 centre (-150.9241, -63.5) radius 7.25
  circle A13 centre (-191.924, -63.5) radius 7.25
  circle A14 centre (-109.926, -63.5) radius 7.25
  circle A15 centre (-68.9244, -63.5) radius 7.25
  circle A16 centre (-0.4322, -38.5669) radius 2.5
  circle A17 centre (-38.4244, -39) radius 25.5
  circle A18 centre (-171.424, -39) radius 15.5
  circle A19 centre (-130.4242, -39) radius 15.5
  circle A20 centre (-89.4244, -39) radius 15.5
  circle A21 centre (-260.424, -39) radius 2.5
  circle A22 centre (-222.424, -39) radius 25.5
  circle A23 centre (-171.4241, -14.5) radius 7.25
  circle A24 centre (-171.4241, -63.5) radius 7.25
  circle A25 centre (-130.4242, -14.5) radius 7.25
  circle A26 centre (-130.425, -63.5) radius 7.25
  line L4 (-68.9244, -14.5) -> (-109.9243, -14.5) construction
  line L5 (-109.926, -63.5) -> (-68.9244, -63.5) construction
  circle A27 centre (-89.4252, -63.5) radius 7.25
  circle A28 centre (-89.4244, -14.5) radius 7.25
  dimension "d102" = 14.5
  dimension "d103" = 14.5
  dimension "d104" = 14.5
  dimension "d105" = 14.5
  dimension "d106" = 14.5
  dimension "d107" = 14.5
  constraint coincident A11.centre L4.start
  constraint coincident A8.centre L4.end
  constraint coincident A14.centre L5.start
  constraint coincident A15.centre L5.end
  constraint midpoint L5 A27.centre
  constraint midpoint L4 A28.centre
  measures "d102" diameter of A23
  measures "d103" diameter of A24
  measures "d104" diameter of A25
  measures "d105" diameter of A26
  measures "d106" diameter of A27
  measures "d107" diameter of A28
extrude "Extrude6" cut sketch "Sketch6" against normal up to surface (10 mm away) contours A23 | A24 | A25 | A26 | A27 | A28 bodies 1 in component "Top_Layer"
move_face "MoveFace14" by (0, -2, 0) 1 faces at (261.0409, 5, -38.1848) on bodies 1 in component "Top_Layer"
move_face "MoveFace15" by (0, -2, 0) 1 faces at (-0.4214, 5, -39.1523) on bodies 1 in component "Top_Layer"
move_face "MoveFace16" to x (1, 0, 0) y (0, 1, 0) z (0, 0, 1) at (0, 0, -3) 3 faces at (82.1842, 3.3333, -63.8614) (135.9789, 3.3333, -68.1602) (164.1831, 3.3333, -63.8614) on bodies 1 in component "Top_Layer"
move_face "MoveFace17" to x (1, 0, 0) y (0, 1, 0) z (0, 0, 1) at (0, 0, 3) 3 faces at (82.1834, 3.3333, -14.8614) (123.1832, 3.3333, -14.8614) (164.1831, 3.3333, -14.8614) on bodies 1 in component "Top_Layer"
move_face "MoveFace14'" by (0, -2, 0) 1 faces at (-0.4214, 5, -39.1523) on bodies 3 in component "Bottom_Layer"
move_face "MoveFace15'" by (0, -2, 0) 1 faces at (261.0409, 5, -38.1848) on bodies 3 in component "Bottom_Layer"
delete_face "DeleteFace2" [no effect] in component "Bottom_Layer"
component "Top_Layer" placed x (1, 0, 0) y (0, 1, 0) z (0, 0, 1) at (10, 0, 0)
component "Bottom_Layer" placed x (1, 0, 0) y (0, 1, 0) z (0, 0, 1) at (10, 0, 0)
